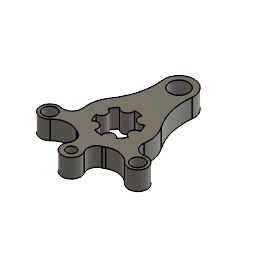
d1.1 (Autodesk Fusion 360 design; units mm, degrees)
part number: 2026-08-05-14-16-29-487
Autodesk Fusion 360 part; units mm, degrees
sketch "Sketch1" plane through (0, 0, 0) normal (0, 1, 0) x (1, 0, 0)
  circle A0 centre (0, 65) radius 10
  circle A1 centre (0, -50) radius 5
  circle A2 centre (-47, -26) radius 7
  arc A3 (-27.0298, 18.9312) -> (-15.8903, 63.1292) centre (-79.4513, 55.6462) ccw
  arc A4 (-44.752, -16.2559) -> (-32.6194, -4.9975) centre (-42.5041, -6.5119) ccw
  arc A5 (-15.6968, -29.0277) -> (-39.7367, -32.8734) centre (-25.21, -46.6203) ccw
  arc A6 (-8.5079, -44.745) -> (-13.0587, -30.3063) centre (-17.0159, -39.49) ccw
  arc A7 (-15.6968, -29.0277) -> (-13.0587, -30.3063) centre (0, 0) ccw
  arc A8 (-27.0298, 18.9312) -> (-32.6194, -4.9975) centre (0, 0) ccw
  arc A9 (15.8903, 63.1292) -> (-15.8903, 63.1292) centre (0, 65) ccw
  arc A10 (-44.752, -16.2559) -> (-39.7367, -32.8734) centre (-47, -26) ccw
  arc A11 (-8.5079, -44.745) -> (8.5079, -44.745) centre (0, -50) ccw
  arc A12 (15.8903, 63.1292) -> (27.0298, 18.9312) centre (79.4513, 55.6462) ccw
  arc A13 (32.6194, -4.9975) -> (27.0298, 18.9312) centre (0, 0) ccw
  arc A14 (32.6194, -4.9975) -> (44.752, -16.2559) centre (42.5041, -6.5119) ccw
  arc A15 (39.7367, -32.8734) -> (44.752, -16.2559) centre (47, -26) ccw
  circle A16 centre (47, -26) radius 7
  arc A17 (39.7367, -32.8734) -> (15.6968, -29.0277) centre (25.21, -46.6203) ccw
  arc A18 (13.0587, -30.3063) -> (15.6968, -29.0277) centre (0, 0) ccw
  arc A19 (13.0587, -30.3063) -> (8.5079, -44.745) centre (17.0159, -39.49) ccw
  arc A20 (-13.27, 14.9635) -> (-2.4581, 19.8484) centre (-8.2346, 18.2261) ccw
  arc A21 (-19.5938, -4.0104) -> (-18.4182, 7.7954) centre (-19.9016, 1.9817) ccw
  arc A22 (-6.3238, -18.9739) -> (-15.9602, -12.0529) centre (-11.667, -16.2444) ccw
  arc A23 (13.27, -14.9635) -> (2.4581, -19.8484) centre (8.2346, -18.2261) ccw
  arc A24 (19.5938, 4.0104) -> (18.4182, -7.7954) centre (19.9016, -1.9817) ccw
  arc A25 (6.3238, 18.9739) -> (15.9602, 12.0529) centre (11.667, 16.2444) ccw
  arc A26 (6.3238, 18.9739) -> (-2.4581, 19.8484) centre (0, 0) ccw
  arc A27 (19.5938, 4.0104) -> (15.9602, 12.0529) centre (0, 0) ccw
  arc A28 (13.27, -14.9635) -> (18.4182, -7.7954) centre (0, 0) ccw
  arc A29 (-6.3238, -18.9739) -> (2.4581, -19.8484) centre (0, 0) ccw
  arc A30 (-13.27, 14.9635) -> (-18.4182, 7.7954) centre (0, 0) ccw
  arc A31 (-19.5938, -4.0104) -> (-15.9602, -12.0529) centre (0, 0) ccw
  dimension "d1" = 66
  dimension "d2" = 40
  dimension "d3" = 32
  dimension "d4" = 20
  dimension "d5" = 65
  dimension "d6" = 20
  dimension "d7" = 10
  dimension "d8" = 14
  dimension "d9" = 20
  dimension "d10" = 26
  dimension "d11" = 24
  dimension "d12" = 47
  dimension "d13" = 128
  dimension "d14" = 20
  dimension "d15" = 40
  dimension "d16" = 20
  dimension "d17" = 12
  dimension "d19" = 360
  constraint coincident A7.centre A8.centre
  constraint concentric A0 A9
  constraint concentric A1 A11
  constraint concentric A2 A10
  constraint tangent A3 A9
  constraint tangent A3 A8
  constraint tangent A4 A10
  constraint tangent A4 A8
  constraint tangent A5 A10
  constraint tangent A5 A7
  constraint tangent A6 A11
  constraint tangent A6 A7
  constraint concentric A7 A8
  constraint coincident A20.centre A30
  constraint concentric A26 A30
  constraint concentric A27 A28
  constraint concentric A28 A29
  constraint concentric A29 A31
  constraint concentric A30 A31
  measures "d1" diameter of A7
  measures "d2" diameter of A30
  measures "d3" diameter of A9
  measures "d4" diameter of A0
  measures "d5" distance of A7.centre A0.centre
  measures "d6" diameter of A11
  measures "d7" diameter of A1
  measures "d8" diameter of A2
  measures "d9" diameter of A10
  measures "d10" vertical distance of A7.centre A2.centre
  measures "d11" vertical distance of A1.centre A2.centre
  measures "d12" horizontal distance of A7.centre A2.centre
  measures "d13" diameter of A3
  measures "d14" diameter of A4
  measures "d15" diameter of A5
  measures "d16" diameter of A6
  measures "d17" diameter of A20
extrude "Extrude1" add sketch "Sketch1" against normal blind 20
